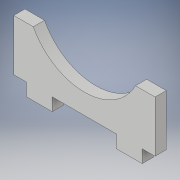
# Autodesk Inventor part: auger_holder
Saved by Autodesk Inventor 2018 (Build 220112000, 112)
## iProperties
Created: 2018-04-09
Part Number: auger_holder
Material: Generic
Document SubType Name: Modeling
Designer: guita
Density: 1 g/cm^3
Appearance: Default
Author: guita
Autodesk Inventor part; units mm, degrees
ref_plane "YZ Plane" through (0, 0, 0) normal (1, 0, 0) x (0, 1, 0)
ref_plane "XZ Plane" through (0, 0, 0) normal (0, 1, 0) x (-1, 0, 0)
ref_plane "XY Plane" through (0, 0, 0) normal (0, 0, 1) x (1, 0, 0)
sketch "Sketch1" plane through (0, 0, 0) normal (0, 0, 1) x (1, 0, 0)
  line L0 (70, 0) -> (70, 25.4)
  line L1 (0, 25.4) -> (0, 0)
  arc A0 (9.6891, 25.4) -> (60.3109, 25.4) centre (35, 38.5) ccw
  line L2 (70, 25.4) -> (60.3109, 25.4)
  line L3 (9.6891, 25.4) -> (0, 25.4)
  line L4 (0, 0) -> (6.35, 0)
  line L5 (6.35, 0) -> (6.35, -6.35)
  line L6 (6.35, -6.35) -> (19.05, -6.35)
  line L7 (19.05, -6.35) -> (19.05, 0)
  line L8 (70, 0) -> (63.65, 0)
  line L9 (63.65, 0) -> (63.65, -6.35)
  line L10 (63.65, -6.35) -> (50.95, -6.35)
  line L11 (50.95, -6.35) -> (50.95, 0)
  line L12 (0, 0) -> (6.35, 0)
  line L13 (19.05, 0) -> (50.95, 0)
  line L14 (63.65, 0) -> (70, 0)
  dimension "d1" = 25.4
  dimension "d6" = 6.35
  dimension "d7" = 12.7
  dimension "d8" = 6.35
  dimension "d9" = 6.35
  dimension "d10" = 12.7
  constraints: 30 end point, 11 perpendicular, 3 horizontal, 2 point on circle, 2 point on line, 1 centre point, 1 parallel
  measures "d1" distance of L0.end L0.start
  measures "d6" distance of L4.end L5.end
  measures "d7" distance of L5.end L6.end
  measures "d8" distance of L0.start L8.end
  measures "d9" distance of L8.end L9.end
  measures "d10" distance of L9.end L10.end
extrude "Extrusion1" add sketch "Sketch1" along normal blind 5.5563
body "Solid1"
